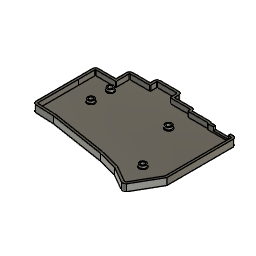
NekoV1 (Autodesk Fusion 360 design; units mm, degrees)
Autodesk Fusion 360 part; units mm, degrees
note: some values were not read from the file. Set by a fixed rule: which sketch regions a step uses.
sketch "Sketch1" plane through (0, 0, 0) normal (0, 0, 1) x (1, 0, 0)
  line L0 (187.7997, -53.8565) -> (167.4907, -53.8666)
  line L1 (94.606, -62.0803) -> (77.4933, -62.0354)
  line L2 (160.6309, -126.1047) -> (174.4556, -134.0879)
  arc A0 (166.5198, -53.1058) -> (167.0103, -53.5064) centre (166.5198, -53.6063) cw
  arc A1 (167.4907, -53.8666) -> (167.0103, -53.5064) centre (167.4907, -53.3661) cw
  line L3 (166.5198, -53.1058) -> (149.4362, -53.1198)
  arc A2 (95.1065, -61.5798) -> (94.606, -62.0803) centre (94.6059, -61.5797) cw
  arc A3 (95.1081, -50.5552) -> (95.6086, -50.0547) centre (95.6086, -50.5552) cw
  line L4 (130.4348, -44.0784) -> (113.6387, -44.0918)
  line L5 (130.9353, -50.1013) -> (130.9353, -44.5789)
  line L6 (148.4352, -50.6175) -> (131.4358, -50.6018)
  line L7 (148.9357, -52.6194) -> (148.9357, -51.1179)
  line L8 (95.1081, -50.5552) -> (95.1065, -61.5798)
  line L9 (112.6549, -50.0547) -> (95.6086, -50.0547)
  line L10 (113.1383, -44.5922) -> (113.1554, -49.5542)
  arc A4 (113.1554, -49.5542) -> (112.6549, -50.0547) centre (112.6549, -49.5542) cw
  arc A5 (113.1383, -44.5922) -> (113.6387, -44.0918) centre (113.6387, -44.5923) cw
  arc A6 (130.4348, -44.0784) -> (130.9353, -44.5789) centre (130.4348, -44.5789) cw
  arc A7 (131.4358, -50.6018) -> (130.9353, -50.1013) centre (131.4358, -50.1013) cw
  arc A8 (148.4352, -50.6175) -> (148.9357, -51.1179) centre (148.4352, -51.1179) cw
  arc A9 (149.4362, -53.1198) -> (148.9357, -52.6194) centre (149.4362, -52.6193) cw
  arc A10 (187.7997, -53.8565) -> (188.3002, -54.357) centre (187.7997, -54.357) cw
  line L11 (94.2226, -113.6087) -> (143.2915, -121.3757)
  arc A11 (175.9364, -133.7828) -> (174.4556, -134.0879) centre (174.8961, -132.4797) cw
  line L12 (77.0866, -93.8666) -> (77.0866, -110.8501)
  line L13 (77.0357, -62.493) -> (77.0866, -76.7815)
  line L14 (188.3002, -54.357) -> (188.3943, -112.1213)
  line L15 (77.0866, -112.223) -> (77.0866, -110.8501)
  line L16 (77.0866, -76.7815) -> (77.0866, -93.8666)
  arc A12 (77.0357, -62.493) -> (77.4933, -62.0354) centre (77.4934, -62.493) cw
  line L17 (77.7476, -112.884) -> (94.2226, -113.6087)
  line L18 (143.2915, -121.3757) -> (160.6309, -126.1047)
  arc A13 (77.7476, -112.884) -> (77.0866, -112.223) centre (77.7476, -112.223) cw
  line L19 (175.9364, -133.7828) -> (188.3943, -112.1213)
  circle A14 centre (95.091, -66.866) radius 2.75
  circle A15 centre (95.091, -66.866) radius 1.75
  circle A16 centre (95.091, -83.9003) radius 2.75
  circle A17 centre (95.091, -83.9003) radius 1.75
  circle A18 centre (149.1137, -69.9169) radius 2.75
  circle A19 centre (149.1137, -69.9169) radius 1.75
  circle A20 centre (167.165, -110.4687) radius 2.75
  circle A21 centre (167.165, -110.4687) radius 1.75
  line L20 (177.5185, -135.0434) -> (190.3951, -112.6539)
  line L21 (190.3002, -54.3554) -> (190.3951, -112.6539)
  arc A22 (190.3002, -54.3554) -> (187.7992, -51.8565) centre (187.7997, -54.357) ccw
  line L22 (187.7992, -51.8565) -> (168.3155, -51.8662)
  arc A23 (168.3155, -51.8662) -> (166.519, -51.1058) centre (166.5198, -53.6063) ccw
  line L23 (166.519, -51.1058) -> (150.9357, -51.1186)
  line L24 (150.9357, -51.1186) -> (150.9357, -51.1179)
  arc A24 (150.9357, -51.1179) -> (148.4369, -48.6175) centre (148.4352, -51.1179) ccw
  line L25 (148.4369, -48.6175) -> (132.9353, -48.6032)
  line L26 (132.9353, -48.6032) -> (132.9353, -44.5789)
  arc A25 (132.9353, -44.5789) -> (130.434, -42.0784) centre (130.4348, -44.5789) ccw
  line L27 (130.434, -42.0784) -> (113.6379, -42.0918)
  arc A26 (113.6379, -42.0918) -> (111.1383, -44.6032) centre (113.6387, -44.5923) ccw
  line L28 (111.1383, -44.6032) -> (111.1502, -48.0547)
  line L29 (111.1502, -48.0547) -> (95.6086, -48.0547)
  arc A27 (95.6086, -48.0547) -> (93.1081, -50.5551) centre (95.6086, -50.5552) ccw
  line L30 (93.1081, -50.5551) -> (93.1067, -60.0763)
  line L31 (93.1067, -60.0763) -> (77.4982, -60.0354)
  arc A28 (77.4982, -60.0354) -> (75.0357, -62.5039) centre (77.4934, -62.493) ccw
  line L32 (75.0357, -62.5039) -> (75.0866, -76.785)
  line L33 (75.0866, -76.785) -> (75.0866, -93.8666)
  line L34 (75.0866, -93.8666) -> (75.0866, -110.8501)
  line L35 (75.0866, -112.223) -> (75.0866, -110.8501)
  arc A29 (75.0866, -112.223) -> (77.6889, -114.8834) centre (77.7476, -112.223) ccw
  line L36 (77.6889, -114.8834) -> (94.0216, -115.6018)
  line L37 (94.0216, -115.6018) -> (142.8708, -123.334)
  line L38 (142.8708, -123.334) -> (159.8549, -127.9661)
  line L39 (159.8549, -127.9661) -> (173.6348, -135.9234)
  arc A30 (173.6348, -135.9234) -> (177.5185, -135.0434) centre (174.8961, -132.4797) ccw
  line L40 (172.1905, -53.8642) -> (185.3472, -53.8642)
  line L41 (185.3472, -53.8642) -> (185.3472, -51.8577)
  line L42 (185.3472, -51.8577) -> (172.1905, -51.8577)
  line L43 (172.1905, -51.8577) -> (172.1905, -53.8642)
  point P0 (95.091, -83.9003)
  point P1 (149.1137, -69.9169)
  point P2 (167.165, -110.4687)
  dimension "d1" = 5.5
  dimension "d2" = 3.5
  dimension "d3" = 5.5
  dimension "d4" = 3.5
  dimension "d5" = 5.5
  dimension "d6" = 3.5
  dimension "d7" = 5.5
  dimension "d8" = 3.5
  dimension "d9" = -2
  constraint coincident P0 A16.centre
  constraint concentric A16 A17
  constraint coincident P1 A18.centre
  constraint coincident P2 A20.centre
  constraint concentric A20 A21
  constraint horizontal L40
  constraint vertical L41
  constraint horizontal L42
  constraint vertical L43
  constraint coincident L22 L41.end
  constraint coincident L0 L40.start
  measures "d1" diameter of A14
  measures "d2" diameter of A15
  measures "d3" diameter of A16
  measures "d4" diameter of A17
  measures "d5" diameter of A18
  measures "d6" diameter of A19
  measures "d7" diameter of A20
  measures "d8" diameter of A21
extrude "Extrude1" add sketch "Sketch1" along normal blind 1.5 contours L0 L1 L2 A0 A1 L3 A2 A3 L4 L5 L6 L7 L8 L9 L10 A4 A5 A6 A7 A8 A9 A10 L11 A11 L12 L13 L14 L15 L16 A12 L17 L18 A13 L19 L40 L41 makes body 1
extrude "Extrude2" add sketch "Sketch1" along normal blind 1 separate body contours A15 makes body 2
extrude "Extrude3" add sketch "Sketch1" along normal blind 1 separate body contours A17 makes body 3
extrude "Extrude4" add sketch "Sketch1" along normal blind 1 separate body contours A19 makes body 4
extrude "Extrude5" add sketch "Sketch1" along normal blind 1 separate body contours A21 makes body 5
extrude "Extrude6" add sketch "Sketch1" along normal blind 4 contours A14 bodies 1 2
extrude "Extrude7" add sketch "Sketch1" along normal blind 4 contours A16 bodies 1 3
extrude "Extrude8" add sketch "Sketch1" along normal blind 4 contours A18 bodies 1 4
extrude "Extrude9" add sketch "Sketch1" along normal blind 4 contours A20 bodies 1 5
extrude "Extrude10" add sketch "Sketch1" along normal blind 6 contours L0 L1 L2 A0 A1 L3 A2 A3 L4 L5 L6 L7 L8 L9 L10 A4 A5 A6 A7 A8 A9 A10 L11 A11 L12 L13 L14 L15 L16 A12 L17 L18 A13 L19 L20 L21 A22 L22 A23 L23 A24 L25 L26 A25 L27 A26 L28 L29 A27 L30 L31 A28 L32 L33 L34 L35 A29 L36 L37 L38 L39 A30 L41 L43 bodies 1
extrude "Extrude11" add sketch "Sketch1" along normal blind 3 contours L0 L22 L41 L43 bodies 1
chamfer "Chamfer1" distance 0.5 angle 45 1 edges at (92.5271, -82.9058, 1.5) on bodies 1
chamfer "Chamfer2" distance 0.5 angle 45 1 edges at (92.5271, -65.8715, 1.5) on bodies 1
chamfer "Chamfer3" distance 0.5 angle 45 1 edges at (146.5498, -68.9225, 1.5) on bodies 1
chamfer "Chamfer4" distance 0.5 angle 45 1 edges at (164.6011, -109.4743, 1.5) on bodies 1
